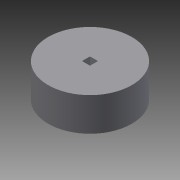
# Autodesk Inventor part: knob
Saved by Autodesk Inventor 2015 (Build 190159000, 159)
## iProperties
Created: 2015-12-08
Part Number: knob
Material: Generic
Document SubType Name: Modeling
Designer: boztalay
Density: 1 g/cm^3
Appearance: Default
Author: boztalay
Autodesk Inventor part; units mm, degrees
ref_plane "YZ Plane" through (0, 0, 0) normal (1, 0, 0) x (0, 1, 0)
ref_plane "XZ Plane" through (0, 0, 0) normal (0, 1, 0) x (-1, 0, 0)
ref_plane "XY Plane" through (0, 0, 0) normal (0, 0, 1) x (1, 0, 0)
sketch "Sketch1" plane through (0, 0, 0) normal (0, 1, 0) x (-1, 0, 0)
  circle A0 centre (0, 0) radius 15.875
  dimension "d0" = 31.75
  constraints: 1 centre point, 1 coincident
  measures "d0" diameter of A0
extrude "Extrusion1" add sketch "Sketch1" along normal blind 12.7
sketch "Sketch4" plane through (0, 0, 0) normal (0, -1, 0) x (1, 0, 0)
  circle A0 centre (0, 0) radius 3.9688
  dimension "d18" = 7.9375
  constraints: 1 centre point, 1 coincident
  measures "d18" diameter of A0
extrude "Extrusion4" add sketch "Sketch4" along normal blind 6.35
sketch "Sketch5" plane through (0, -6.35, 0) normal (0, -1, 0) x (1, 0, 0)
  line L0 (1.524, 1.524) -> (-1.524, 1.524)
  line L1 (-1.524, 1.524) -> (-1.524, -1.524)
  line L2 (-1.524, -1.524) -> (1.524, -1.524)
  line L3 (1.524, -1.524) -> (1.524, 1.524)
  line L4 (1.524, 1.524) -> (-1.524, -1.524) construction
  line L5 (-1.524, 1.524) -> (1.524, -1.524) construction
  point P0 (0, 0)
  dimension "d21" = 3.048
  constraints: 12 end point, 2 midpoint, 2 parallel, 2 perpendicular, 1 horizontal
  measures "d21" distance of L0.end L1.end
extrude "Extrusion5" cut sketch "Sketch5" against normal blind 19.05
body "Solid1"
